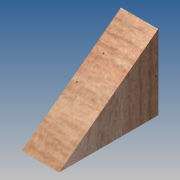
# Autodesk Inventor part: endBlock
Saved by Autodesk Inventor 2014 SP1 (Build 180222100, 222)
## iProperties
Created: 2014-08-18
Part Number: endBlock
Material: Wood (Birch)
Document SubType Name: Modeling
Designer: Dave
Mass: 116.961 g
Surface Area: 251.011 cm^2
Volume: 212.655 cm^3
Density: 0.55 g/cm^3
Appearance: Birch - Natural Polished
Author: Dave
Autodesk Inventor part; units mm, degrees
ref_plane "YZ Plane" through (0, 0, 0) normal (1, 0, 0) x (0, 1, 0)
ref_plane "XZ Plane" through (0, 0, 0) normal (0, 1, 0) x (-1, 0, 0)
ref_plane "XY Plane" through (0, 0, 0) normal (0, 0, 1) x (1, 0, 0)
sketch "Sketch1" plane through (0, 0, 0) normal (1, 0, 0) x (0, 1, 0)
  line L0 (0, 0) -> (76.4305, -101.4267)
  line L1 (0, 0) -> (127, 0) construction
  line L2 (76.4305, -101.4267) -> (0, -101.4267)
  line L3 (0, -101.4267) -> (0, 0)
  dimension "d0" = 127
  dimension "d1" = 53
  constraints: 8 end point, 2 horizontal, 1 equal length, 1 perpendicular
  measures "d0" distance of L0.start L0.end
  measures "d1" angle of L0 L1
extrude "Extrusion1" add sketch "Sketch1" along normal blind 38.1
body "Solid1"
